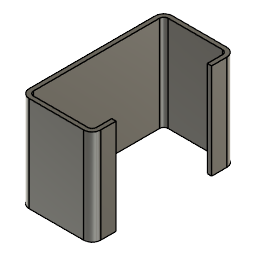
RC-150×75×25×4.5 (Autodesk Fusion 360 design; units mm, degrees)
Autodesk Fusion 360 part; units mm, degrees
sketch "スケッチ1" plane through (0, 0, 0) normal (0, 0, 1) x (1, 0, 0)
  line L0 (65.6268, -79.7784) -> (8.6268, -79.7784)
  line L1 (8.6268, -75.2784) -> (65.6268, -75.2784)
  line L2 (8.6268, 65.7216) -> (65.6268, 65.7216)
  line L3 (8.6268, 70.2216) -> (65.6268, 70.2216)
  line L4 (4.1268, 61.2216) -> (4.1268, -70.7784)
  line L5 (-0.3732, 61.2216) -> (-0.3732, -70.7784)
  arc A0 (-0.3732, -70.7784) -> (8.6268, -79.7784) centre (8.6268, -70.7784) ccw
  arc A1 (4.1268, -70.7784) -> (8.6268, -75.2784) centre (8.6268, -70.7784) ccw
  arc A2 (8.6268, 70.2216) -> (-0.3732, 61.2216) centre (8.6268, 61.2216) ccw
  arc A3 (8.6268, 65.7216) -> (4.1268, 61.2216) centre (8.6268, 61.2216) ccw
  line L6 (70.1268, -70.7784) -> (70.1268, -54.7784)
  line L7 (74.6268, -70.7784) -> (74.6268, -54.7784)
  arc A4 (65.6268, -79.7784) -> (74.6268, -70.7784) centre (65.6268, -70.7784) ccw
  arc A5 (65.6268, -75.2784) -> (70.1268, -70.7784) centre (65.6268, -70.7784) ccw
  line L8 (74.6268, -54.7784) -> (70.1268, -54.7784)
  line L9 (74.6268, 61.2216) -> (74.6268, 45.2216)
  line L10 (70.1268, 61.2216) -> (70.1268, 45.2216)
  line L11 (70.1268, 45.2216) -> (74.6268, 45.2216)
  arc A6 (74.6268, 61.2216) -> (65.6268, 70.2216) centre (65.6268, 61.2216) ccw
  arc A7 (70.1268, 61.2216) -> (65.6268, 65.7216) centre (65.6268, 61.2216) ccw
  point P0 (-0.3732, 70.2216)
extrude "押し出し1" add sketch "スケッチ1" along normal blind 100
